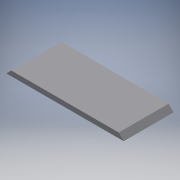
# Autodesk Inventor part: deksel token
Saved by Autodesk Inventor 2018 (Build 220112000, 112)
## iProperties
Created: 2020-11-30
Part Number: deksel token
Material: Generic
Document SubType Name: Modeling
Designer: Olivi
Density: 1 g/cm^3
Appearance: Default
Author: Olivi
## iProperties of the stored document deksel token_3DPrint.ipt
Created: 2020-12-04
Part Number: deksel token_3DPrint
Material: Generic
Document SubType Name: Modeling
Designer: Olivi
Density: 1 g/cm^3
Appearance: Default
Author: Olivi
Autodesk Inventor part; units mm, degrees
ref_plane "YZ Plane" through (0, 0, 0) normal (1, 0, 0) x (0, 1, 0)
ref_plane "XZ Plane" through (0, 0, 0) normal (0, 1, 0) x (-1, 0, 0)
ref_plane "XY Plane" through (0, 0, 0) normal (0, 0, 1) x (1, 0, 0)
sketch "Sketch1" plane through (0, 0, 0) normal (0, 0, 1) x (1, 0, 0)
  line L0 (0, 0) -> (43, 0)
  line L1 (43, 0) -> (43, 20)
  line L2 (43, 20) -> (0, 20)
  line L3 (0, 20) -> (0, 0)
  dimension "d0" = 43
  dimension "d1" = 20
  constraints: 8 end point, 2 parallel, 1 horizontal, 1 perpendicular
  measures "d0" distance of L2.end L1.end
  measures "d1" distance of L1.end L0.end
extrude "Extrusion1" add sketch "Sketch1" along normal blind 2
sketch "Sketch2" plane through (0, 0, 0) normal (0, -1, 0) x (1, 0, 0)
  line L0 (43, 0) -> (43, 2) projected
  line L1 (0, 0) -> (0, 2) projected
  line L2 (0, 0) -> (-2, 0)
  line L3 (-2, 0) -> (0, 2)
  line L4 (43, 0) -> (45, 0)
  line L5 (45, 0) -> (43, 2)
  dimension "d4" = 2
  dimension "d5" = 2
  constraints: 8 end point, 2 horizontal
  measures "d4" distance of L1.start L2.end
  measures "d5" distance of L0.start L4.end
extrude "Extrusion2" add sketch "Sketch2" against normal blind 20
body "Solid1"
